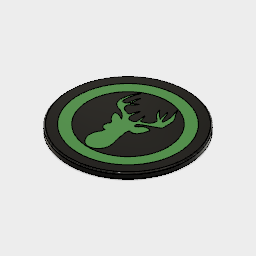
DeerHeadSaucer v4 (Autodesk Fusion 360 design; units mm, degrees)
Autodesk Fusion 360 part; units mm, degrees
sketch "Sketch1" plane through (0, 0, 0) normal (0, 1, 0) x (1, 0, 0)
  circle A0 centre (0, 0) radius 45
  dimension "d1" = 90
  measures "d1" diameter of A0
sketch "Sketch2" plane through (0, 5, 0) normal (0, 1, 0) x (-1, 0, 0)
  circle A0 centre (0, 0) radius 45
  circle A1 centre (0, 0) radius 37.5
  circle A2 centre (0, 0) radius 30
  circle A3 centre (0, 0) radius 45
  dimension "d4" = 75
  dimension "d5" = 60
  measures "d4" diameter of A1
  measures "d5" diameter of A2
extrude "Extrude12" add sketch "Sketch2" against normal blind 5 contours A2 makes body 1
extrude "Extrude5" add sketch "Sketch2" against normal blind 5 separate body contours A0 A3 makes body 2
extrude "Extrude8" add sketch "Sketch2" against normal blind 5 separate body contours A1 makes body 3
fillet "Fillet1" radius 1 2 edges at (41.9547, 0, 16.2727) (41.9547, 5, -16.2727) on bodies 2
sketch "Sketch3" plane through (0, 5, 0) normal (0, 1, 0) x (-1, 0, 0)
  circle A0 centre (0, 0) radius 30
  spline S0 degree 3 poles (5.3201, 12.0156) (5.6403, 11.9964) (5.9225, 11.9623) (6.2042, 11.9659) knots 0 0 0 0 1 1 1 1
  spline S1 degree 3 poles (6.2042, 11.9659) (6.9405, 11.9753) (7.4513, 11.6333) (7.7836, 10.9942) knots 0 0 0 0 1 1 1 1
  spline S2 degree 3 poles (7.7836, 10.9942) (7.814, 10.9357) (7.8257, 10.8444) (7.8725, 10.8212) knots 0 0 0 0 1 1 1 1
  spline S3 degree 3 poles (7.8725, 10.8212) (9.2801, 10.1198) (8.7297, 8.8499) (8.6485, 7.8037) knots 0 0 0 0 1 1 1 1
  spline S4 degree 3 poles (8.6485, 7.8037) (8.6004, 7.1844) (8.1656, 6.568) (7.813, 6.008) knots 0 0 0 0 1 1 1 1
  spline S5 degree 3 poles (7.813, 6.008) (7.5196, 5.542) (7.5763, 4.6327) (8.0375, 4.3382) knots 0 0 0 0 1 1 1 1
  spline S6 degree 3 poles (8.0375, 4.3382) (10.1616, 2.9821) (11.3332, 0.8983) (12.2794, -1.3264) knots 0 0 0 0 1 1 1 1
  spline S7 degree 3 poles (12.2794, -1.3264) (12.7209, -2.3645) (12.2531, -2.9451) (11.1174, -2.9054) knots 0 0 0 0 1 1 1 1
  spline S8 degree 3 poles (11.1174, -2.9054) (9.6288, -2.8534) (8.2885, -2.326) (7.0385, -1.5411) knots 0 0 0 0 1 1 1 1
  spline S9 degree 3 poles (7.0385, -1.5411) (6.7437, -1.356) (6.4395, -1.1863) (6.0249, -1.0832) knots 0 0 0 0 1 1 1 1
  spline S10 degree 3 poles (6.0249, -1.0832) (6.125, -1.2787) (6.2066, -1.4867) (6.328, -1.668) knots 0 0 0 0 1 1 1 1
  spline S11 degree 3 poles (6.328, -1.668) (7.8418, -3.9288) (10.0065, -5.3484) (12.4664, -6.3718) knots 0 0 0 0 1 1 1 1
  spline S12 degree 3 poles (12.4664, -6.3718) (13.276, -6.7087) (14.1223, -6.958) (14.9298, -7.2992) knots 0 0 0 0 1 1 1 1
  spline S13 degree 3 poles (14.9298, -7.2992) (17.9946, -8.5941) (19.4228, -11.0862) (19.0776, -14.4106) knots 0 0 0 0 1 1 1 1
  spline S14 degree 3 poles (19.0776, -14.4106) (18.754, -17.5276) (17.9758, -20.5015) (16.396, -23.2308) knots 0 0 0 0 1 1 1 1
  spline S15 degree 3 poles (16.396, -23.2308) (16.0797, -23.7774) (15.696, -24.2849) (15.1985, -24.7419) knots 0 0 0 0 1 1 1 1
  spline S16 degree 3 poles (15.1985, -24.7419) (15.32, -24.39) (15.4319, -24.0345) (15.5645, -23.6868) knots 0 0 0 0 1 1 1 1
  spline S17 degree 3 poles (15.5645, -23.6868) (16.7111, -20.6835) (17.4507, -17.604) (17.3276, -14.361) knots 0 0 0 0 1 1 1 1
  spline S18 degree 3 poles (17.3276, -14.361) (17.3243, -14.2728) (17.3256, -14.1844) (17.3177, -14.0968) knots 0 0 0 0 1 1 1 1
  spline S19 degree 3 poles (17.3177, -14.0968) (17.1612, -12.363) (16.7765, -12.1575) (15.1959, -12.7756) knots 0 0 0 0 1 1 1 1
  spline S20 degree 3 poles (15.1959, -12.7756) (14.1702, -13.1766) (13.6603, -13.6929) (13.6995, -14.9268) knots 0 0 0 0 1 1 1 1
  spline S21 degree 3 poles (13.6995, -14.9268) (13.7655, -17.007) (13.2058, -19.0149) (12.4005, -20.9388) knots 0 0 0 0 1 1 1 1
  spline S22 degree 3 poles (12.4005, -20.9388) (12.3048, -21.1674) (12.1686, -21.3789) (11.9551, -21.5523) knots 0 0 0 0 1 1 1 1
  spline S23 degree 3 poles (11.9551, -21.5523) (12.2245, -19.1461) (12.4938, -16.7399) (12.7633, -14.3337) knots 0 0 0 0 1 1 1 1
  spline S24 degree 3 poles (12.7633, -14.3337) (12.693, -14.285) (12.6229, -14.2362) (12.5527, -14.1875) knots 0 0 0 0 1 1 1 1
  spline S25 degree 3 poles (12.5527, -14.1875) (11.309, -15.1894) (10.0654, -16.1913) (8.8217, -17.1933) knots 0 0 0 0 1 1 1 1
  spline S26 degree 3 poles (8.8217, -17.1933) (8.7861, -17.171) (8.7505, -17.1488) (8.715, -17.1266) knots 0 0 0 0 1 1 1 1
  spline S27 degree 3 poles (8.715, -17.1266) (8.8305, -16.8849) (8.9189, -16.6253) (9.066, -16.4048) knots 0 0 0 0 1 1 1 1
  spline S28 degree 3 poles (9.066, -16.4048) (9.9271, -15.1129) (10.9296, -13.9487) (12.2346, -13.0827) knots 0 0 0 0 1 1 1 1
  spline S29 degree 3 poles (12.2346, -13.0827) (12.5823, -12.8519) (12.7649, -12.5955) (12.7073, -12.1642) knots 0 0 0 0 1 1 1 1
  spline S30 degree 3 poles (12.7073, -12.1642) (12.6345, -11.6203) (12.6305, -11.0659) (12.5388, -10.5259) knots 0 0 0 0 1 1 1 1
  spline S31 degree 3 poles (12.5388, -10.5259) (12.3364, -9.3341) (11.6126, -8.5675) (10.4962, -8.148) knots 0 0 0 0 1 1 1 1
  spline S32 degree 3 poles (10.4962, -8.148) (9.5099, -7.7773) (8.5287, -7.3926) (7.5379, -7.0344) knots 0 0 0 0 1 1 1 1
  spline S33 degree 3 poles (7.5379, -7.0344) (6.5038, -6.6606) (6.3039, -6.7819) (5.9223, -7.792) knots 0 0 0 0 1 1 1 1
  spline S34 degree 3 poles (5.9223, -7.792) (5.3562, -9.291) (4.7596, -10.7788) (4.1681, -12.2683) knots 0 0 0 0 1 1 1 1
  spline S35 degree 3 poles (4.1681, -12.2683) (4.0897, -12.4656) (3.9649, -12.6444) (3.8614, -12.8318) knots 0 0 0 0 1 1 1 1
  spline S36 degree 3 poles (3.8614, -12.8318) (3.7968, -12.8197) (3.7321, -12.8076) (3.6674, -12.7955) knots 0 0 0 0 1 1 1 1
  spline S37 degree 3 poles (3.6674, -12.7955) (3.708, -12.435) (3.7378, -12.0729) (3.7912, -11.7142) knots 0 0 0 0 1 1 1 1
  spline S38 degree 3 poles (3.7912, -11.7142) (4.0235, -10.1554) (4.3606, -8.6043) (4.4673, -7.0373) knots 0 0 0 0 1 1 1 1
  spline S39 degree 3 poles (4.4673, -7.0373) (4.5477, -5.8564) (4.1261, -4.7248) (3.2438, -3.8663) knots 0 0 0 0 1 1 1 1
  spline S40 degree 3 poles (3.2438, -3.8663) (3.005, -3.6339) (2.6135, -3.4746) (2.2776, -3.4445) knots 0 0 0 0 1 1 1 1
  spline S41 degree 3 poles (2.2776, -3.4445) (1.713, -3.394) (1.1304, -3.4292) (0.5665, -3.508) knots 0 0 0 0 1 1 1 1
  spline S42 degree 3 poles (0.5665, -3.508) (-0.6773, -3.6819) (-1.5171, -4.6047) (-1.4715, -5.8514) knots 0 0 0 0 1 1 1 1
  spline S43 degree 3 poles (-1.4715, -5.8514) (-1.4307, -6.9679) (-1.2372, -8.0783) (-1.1281, -9.193) knots 0 0 0 0 1 1 1 1
  spline S44 degree 3 poles (-1.1281, -9.193) (-1.0504, -9.9862) (-1.0007, -10.782) (-0.9386, -11.5767) knots 0 0 0 0 1 1 1 1
  spline S45 degree 3 poles (-0.9386, -11.5767) (-1.0236, -11.5919) (-1.1084, -11.6069) (-1.1934, -11.6221) knots 0 0 0 0 1 1 1 1
  spline S46 degree 3 poles (-1.1934, -11.6221) (-1.364, -11.1374) (-1.5627, -10.6604) (-1.6995, -10.1662) knots 0 0 0 0 1 1 1 1
  spline S47 degree 3 poles (-1.6995, -10.1662) (-1.9687, -9.193) (-2.1888, -8.2061) (-2.4578, -7.2327) knots 0 0 0 0 1 1 1 1
  spline S48 degree 3 poles (-2.4578, -7.2327) (-2.6736, -6.4513) (-2.9181, -6.2972) (-3.6471, -6.625) knots 0 0 0 0 1 1 1 1
  spline S49 degree 3 poles (-3.6471, -6.625) (-4.8044, -7.1452) (-5.9723, -7.6709) (-7.0472, -8.3371) knots 0 0 0 0 1 1 1 1
  spline S50 degree 3 poles (-7.0472, -8.3371) (-8.2315, -9.0711) (-8.6485, -10.3242) (-8.8493, -11.6475) knots 0 0 0 0 1 1 1 1
  spline S51 degree 3 poles (-8.8493, -11.6475) (-9.1024, -13.3154) (-9.0999, -13.3099) (-7.6536, -14.1641) knots 0 0 0 0 1 1 1 1
  spline S52 degree 3 poles (-7.6536, -14.1641) (-5.1039, -15.6701) (-3.6845, -18.0166) (-2.787, -20.7458) knots 0 0 0 0 1 1 1 1
  spline S53 degree 3 poles (-2.787, -20.7458) (-2.7622, -20.821) (-2.7839, -20.9117) (-2.8515, -21.0493) knots 0 0 0 0 1 1 1 1
  spline S54 degree 3 poles (-2.8515, -21.0493) (-4.4103, -18.7466) (-6.4739, -17.0079) (-8.7276, -15.4758) knots 0 0 0 0 1 1 1 1
  spline S55 degree 3 poles (-8.7276, -15.4758) (-8.7899, -15.5024) (-8.8524, -15.529) (-8.9147, -15.5555) knots 0 0 0 0 1 1 1 1
  spline S56 degree 3 poles (-8.9147, -15.5555) (-8.3289, -17.8598) (-7.7433, -20.1641) (-7.1575, -22.4685) knots 0 0 0 0 1 1 1 1
  spline S57 degree 3 poles (-7.1575, -22.4685) (-7.2269, -22.5046) (-7.2963, -22.5407) (-7.3658, -22.5768) knots 0 0 0 0 1 1 1 1
  spline S58 degree 3 poles (-7.3658, -22.5768) (-7.5627, -22.314) (-7.8247, -22.0781) (-7.946, -21.7841) knots 0 0 0 0 1 1 1 1
  spline S59 degree 3 poles (-7.946, -21.7841) (-8.7814, -19.7582) (-9.6717, -17.7482) (-10.3608, -15.6721) knots 0 0 0 0 1 1 1 1
  spline S60 degree 3 poles (-10.3608, -15.6721) (-10.6326, -14.8531) (-11.0466, -14.546) (-11.8258, -14.4077) knots 0 0 0 0 1 1 1 1
  spline S61 degree 3 poles (-11.8258, -14.4077) (-12.4042, -16.1873) (-12.102, -17.9692) (-11.8511, -19.7386) knots 0 0 0 0 1 1 1 1
  spline S62 degree 3 poles (-11.8511, -19.7386) (-11.602, -21.4942) (-11.4867, -23.3082) (-10.0856, -24.6893) knots 0 0 0 0 1 1 1 1
  spline S63 degree 3 poles (-10.0856, -24.6893) (-10.1691, -24.6998) (-10.2526, -24.7104) (-10.3361, -24.7209) knots 0 0 0 0 1 1 1 1
  spline S64 degree 3 poles (-10.3361, -24.7209) (-10.3613, -24.8957) (-10.4533, -25.0947) (-10.4005, -25.2414) knots 0 0 0 0 1 1 1 1
  spline S65 degree 3 poles (-10.4005, -25.2414) (-10.1388, -25.9674) (-9.8389, -26.6795) (-9.5525, -27.3966) knots 0 0 0 0 1 1 1 1
  spline S66 degree 3 poles (-9.5525, -27.3966) (-9.6376, -27.4369) (-9.7229, -27.4774) (-9.8081, -27.5178) knots 0 0 0 0 1 1 1 1
  spline S67 degree 3 poles (-9.8081, -27.5178) (-10.4171, -26.4363) (-11.0145, -25.3482) (-11.6405, -24.2767) knots 0 0 0 0 1 1 1 1
  spline S68 degree 3 poles (-11.6405, -24.2767) (-11.9024, -23.8282) (-12.1635, -23.3523) (-12.5297, -22.9965) knots 0 0 0 0 1 1 1 1
  spline S69 degree 3 poles (-12.5297, -22.9965) (-14.3373, -21.2394) (-15.2978, -19.1044) (-15.4313, -16.6071) knots 0 0 0 0 1 1 1 1
  spline S70 degree 3 poles (-15.4313, -16.6071) (-15.5249, -14.8543) (-15.5532, -13.0977) (-15.5832, -11.3422) knots 0 0 0 0 1 1 1 1
  spline S71 degree 3 poles (-15.5832, -11.3422) (-15.5966, -10.557) (-15.251, -9.9594) (-14.5308, -9.5778) knots 0 0 0 0 1 1 1 1
  spline S72 degree 3 poles (-14.5308, -9.5778) (-11.8712, -8.1683) (-9.2131, -6.7558) (-6.5677, -5.3202) knots 0 0 0 0 1 1 1 1
  spline S73 degree 3 poles (-6.5677, -5.3202) (-5.8166, -4.9126) (-5.0938, -4.4464) (-4.3886, -3.9625) knots 0 0 0 0 1 1 1 1
  spline S74 degree 3 poles (-4.3886, -3.9625) (-3.7593, -3.5307) (-3.4131, -2.8878) (-3.3395, -2.1322) knots 0 0 0 0 1 1 1 1
  spline S75 degree 3 poles (-3.3395, -2.1322) (-3.3148, -1.8782) (-3.3579, -1.4662) (-3.5113, -1.3809) knots 0 0 0 0 1 1 1 1
  spline S76 degree 3 poles (-3.5113, -1.3809) (-3.7568, -1.2446) (-4.1534, -1.2306) (-4.4254, -1.3302) knots 0 0 0 0 1 1 1 1
  spline S77 degree 3 poles (-4.4254, -1.3302) (-4.7609, -1.4531) (-5.0574, -1.7207) (-5.3287, -1.9711) knots 0 0 0 0 1 1 1 1
  spline S78 degree 3 poles (-5.3287, -1.9711) (-5.6511, -2.2687) (-5.9523, -2.5963) (-6.2223, -2.9425) knots 0 0 0 0 1 1 1 1
  spline S79 degree 3 poles (-6.2223, -2.9425) (-7.6053, -4.7157) (-9.4782, -4.9419) (-11.5172, -4.6308) knots 0 0 0 0 1 1 1 1
  spline S80 degree 3 poles (-11.5172, -4.6308) (-12.0475, -4.5499) (-12.3742, -4.2062) (-12.277, -3.6592) knots 0 0 0 0 1 1 1 1
  spline S81 degree 3 poles (-12.277, -3.6592) (-11.8348, -1.1695) (-11.181, 1.2521) (-9.3162, 3.1007) knots 0 0 0 0 1 1 1 1
  spline S82 degree 3 poles (-9.3162, 3.1007) (-8.8556, 3.5572) (-8.1795, 3.8583) (-7.5478, 4.0584) knots 0 0 0 0 1 1 1 1
  spline S83 degree 3 poles (-7.5478, 4.0584) (-7.138, 4.1882) (-6.5879, 4.1082) (-6.1736, 3.9411) knots 0 0 0 0 1 1 1 1
  spline S84 degree 3 poles (-6.1736, 3.9411) (-5.3662, 3.6154) (-4.8423, 3.7065) (-4.6319, 4.5754) knots 0 0 0 0 1 1 1 1
  spline S85 degree 3 poles (-4.6319, 4.5754) (-4.4518, 5.319) (-4.4449, 6.1456) (-4.5507, 6.9092) knots 0 0 0 0 1 1 1 1
  spline S86 degree 3 poles (-4.5507, 6.9092) (-4.8037, 8.7345) (-5.2275, 10.5364) (-5.4695, 12.3627) knots 0 0 0 0 1 1 1 1
  spline S87 degree 3 poles (-5.4695, 12.3627) (-5.6697, 13.8749) (-6.0732, 15.3078) (-6.5179, 16.7644) knots 0 0 0 0 1 1 1 1
  spline S88 degree 3 poles (-6.5179, 16.7644) (-7.2556, 19.1804) (-7.548, 21.7023) (-6.5831, 24.1458) knots 0 0 0 0 1 1 1 1
  spline S89 degree 3 poles (-6.5831, 24.1458) (-5.5576, 26.7425) (-3.6413, 28.4588) (-0.9313, 29.1581) knots 0 0 0 0 1 1 1 1
  spline S90 degree 3 poles (-0.9313, 29.1581) (1.6662, 29.8285) (4.4632, 28.5946) (6.1576, 26.1653) knots 0 0 0 0 1 1 1 1
  spline S91 degree 3 poles (6.1576, 26.1653) (8.4383, 22.8955) (8.403, 18.3229) (5.8952, 14.9154) knots 0 0 0 0 1 1 1 1
  spline S92 degree 3 poles (5.8952, 14.9154) (5.1822, 13.9465) (5.2706, 13.0469) (5.3201, 12.0156) knots 0 0 0 0 1 1 1 1
  spline S93 degree 3 poles (13.6169, -9.2714) (13.6846, -10.278) (13.7392, -11.0903) (13.7988, -11.9766) knots 0 0 0 0 1 1 1 1
  spline S94 degree 3 poles (13.7988, -11.9766) (14.4546, -11.5701) (15.0359, -11.2096) (15.7669, -10.7566) knots 0 0 0 0 1 1 1 1
  spline S95 degree 3 poles (15.7669, -10.7566) (15.0025, -10.2287) (14.3686, -9.7907) (13.6169, -9.2714) knots 0 0 0 0 1 1 1 1
  spline S96 degree 3 poles (-13.5746, -14.4204) (-14.4268, -15.0897) (-14.161, -18.634) (-13.159, -19.98) knots 0 0 0 0 1 1 1 1
  spline S97 degree 3 poles (-13.159, -19.98) (-13.2954, -18.156) (-13.4358, -16.2768) (-13.5746, -14.4204) knots 0 0 0 0 1 1 1 1
  spline S98 degree 3 poles (-10.547, -10.9728) (-11.2168, -11.3905) (-11.5788, -11.8321) (-11.4767, -12.3565) knots 0 0 0 0 1 1 1 1
  spline S99 degree 3 poles (-11.4767, -12.3565) (-11.4263, -12.6154) (-10.8966, -12.781) (-10.5838, -12.9888) knots 0 0 0 0 1 1 1 1
  spline S100 degree 3 poles (-10.5838, -12.9888) (-10.5304, -12.9447) (-10.477, -12.9006) (-10.4236, -12.8564) knots 0 0 0 0 1 1 1 1
  spline S101 degree 3 poles (-10.4236, -12.8564) (-10.4611, -12.2835) (-10.4987, -11.7107) (-10.547, -10.9728) knots 0 0 0 0 1 1 1 1
extrude "Extrude13" cut sketch "Sketch3" against normal blind 5 contours S0 S1 S2 S3 S4 S5 S6 S7 S8 S9 S10 S11 S12 S13 S14 S15 S16 S17 S18 S19 S20 S21 S22 S23 S24 S25 S26 S27 S28 S29 S30 S31 S32 S33 S34 S35 S36 S37 S38 S39 S40 S41 S42 S43 S44 S45 S46 S47 S48 S49 S50 S51 S52 S53 S54 S55 S56 S57 S58 S59 S60 S61 S62 S63 S64 S65 S66 S67 S68 S69 S70 S71 S72 S73 S74 S75 S76 S77 S78 S79 S80 S81 S82 S83 S84 S85 S86 S87 S88 S89 S90 S91 S92 | S93 S94 S95 | S96 S97 | S98 S99 S100 S101 bodies 1
extrude "Extrude14" add sketch "Sketch3" against normal blind 5 separate body contours S0 S1 S2 S3 S4 S5 S6 S7 S8 S9 S10 S11 S12 S13 S14 S15 S16 S17 S18 S19 S20 S21 S22 S23 S24 S25 S26 S27 S28 S29 S30 S31 S32 S33 S34 S35 S36 S37 S38 S39 S40 S41 S42 S43 S44 S45 S46 S47 S48 S49 S50 S51 S52 S53 S54 S55 S56 S57 S58 S59 S60 S61 S62 S63 S64 S65 S66 S67 S68 S69 S70 S71 S72 S73 S74 S75 S76 S77 S78 S79 S80 S81 S82 S83 S84 S85 S86 S87 S88 S89 S90 S91 S92 | S93 S94 S95 | S96 S97 | S98 S99 S100 S101 makes body 4
copy_body "Body->Comp8" bodies 4 removing the originals makes body 5 in component "DeerHead"
copy_body "Body->Comp9" bodies 1 removing the originals makes body 6 in component "DeerHeadPlate"
copy_body "Body->Comp10" bodies 2 removing the originals makes body 7 in component "OuterRing"
copy_body "Body->Comp11" bodies 3 removing the originals makes body 8 in component "InnerRing"
component "DeerHead" placed x (1, 0, 0) y (0, 1, 0) z (0, 0, 1) at (0, 0, 0)
component "DeerHeadPlate" placed x (1, 0, 0) y (0, 1, 0) z (0, 0, 1) at (0, 0, 0)
component "OuterRing" placed x (1, 0, 0) y (0, 1, 0) z (0, 0, 1) at (0, 0, 0)
component "InnerRing" placed x (1, 0, 0) y (0, 1, 0) z (0, 0, 1) at (0, 0, 0)
named bodies: "OuterRing", "InnerRing", "DearHeadPlate", "DearHead"
